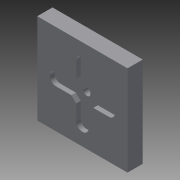
# Autodesk Inventor part: ServoArmTrace
Saved by Autodesk Inventor 2014 (Build 180170000, 170)
## iProperties
Created: 2013-09-20
Part Number: ServoArmTrace
Material: Generic
Document SubType Name: Modeling
Designer: Medrimonia
Density: 1 g/cm^3
Appearance: Default
Author: Medrimonia
Autodesk Inventor part; units mm, degrees
ref_plane "YZ Plane" through (0, 0, 0) normal (1, 0, 0) x (0, 1, 0)
ref_plane "XZ Plane" through (0, 0, 0) normal (0, 1, 0) x (-1, 0, 0)
ref_plane "XY Plane" through (0, 0, 0) normal (0, 0, 1) x (1, 0, 0)
sketch "Sketch1" plane through (0, 0, 0) normal (0, 1, 0) x (-1, 0, 0)
  line L0 (-18.95, -18.95) -> (18.95, -18.95)
  line L1 (18.95, -18.95) -> (18.95, 18.95)
  line L2 (18.95, 18.95) -> (-18.95, 18.95)
  line L3 (-18.95, 18.95) -> (-18.95, -18.95)
  line L4 (-18.95, -18.95) -> (18.95, 18.95) construction
  line L5 (18.95, -18.95) -> (-18.95, 18.95) construction
  line L6 (-2.45, -13.45) -> (2.45, -13.45) construction
  line L7 (2.45, -13.45) -> (2.45, 13.45) construction
  line L8 (2.45, 13.45) -> (-2.45, 13.45) construction
  line L9 (-2.45, 13.45) -> (-2.45, -13.45) construction
  line L10 (-2.45, -13.45) -> (2.45, 13.45) construction
  line L11 (2.45, -13.45) -> (-2.45, 13.45) construction
  line L12 (-13.45, -2.45) -> (13.45, -2.45) construction
  line L13 (13.45, -2.45) -> (13.45, 2.45) construction
  line L14 (13.45, 2.45) -> (-13.45, 2.45) construction
  line L15 (-13.45, 2.45) -> (-13.45, -2.45) construction
  line L16 (-13.45, -2.45) -> (13.45, 2.45) construction
  line L17 (13.45, -2.45) -> (-13.45, 2.45) construction
  line L18 (-13.6, -2.6) -> (13.6, -2.6)
  line L19 (13.6, -2.6) -> (13.6, 2.6)
  line L20 (13.6, 2.6) -> (-13.6, 2.6)
  line L21 (-13.6, 2.6) -> (-13.6, -2.6)
  line L22 (-13.6, -2.6) -> (13.6, 2.6) construction
  line L23 (13.6, -2.6) -> (-13.6, 2.6) construction
  line L24 (-2.6, -13.6) -> (2.6, -13.6)
  line L25 (2.6, -13.6) -> (2.6, 13.6)
  line L26 (2.6, 13.6) -> (-2.6, 13.6)
  line L27 (-2.6, 13.6) -> (-2.6, -13.6)
  line L28 (-2.6, -13.6) -> (2.6, 13.6) construction
  line L29 (2.6, -13.6) -> (-2.6, 13.6) construction
  point P0 (0, 0)
  point P1 (0, 0)
  dimension "d0" = 37.9
  dimension "d1" = 4.9
  dimension "d2" = 11
  dimension "d3" = 0.15
  dimension "d4" = 0.15
  constraints: 60 end point, 12 midpoint, 10 parallel, 10 perpendicular, 5 horizontal
  measures "d0" distance of L1.end L2.end
  measures "d1" distance of L14.end L12.start
  measures "d2" distance between parallel lines of L13 L7
  measures "d3" distance between parallel lines of L25 L7
  measures "d4" distance between parallel lines of L26 L8
extrude "Extrusion1" add sketch "Sketch1" along normal blind 1.9
sketch "Sketch2" plane through (0, 1.9, 0) normal (0, 1, 0) x (1, 0, 0)
  line L0 (18.95, 18.95) -> (-18.95, 18.95) projected
  line L1 (-18.95, 18.95) -> (-18.95, -18.95) projected
  line L2 (-18.95, -18.95) -> (18.95, -18.95) projected
  line L3 (18.95, -18.95) -> (18.95, 18.95) projected
  circle A0 centre (0, 0) radius 1.5
  dimension "d7" = 3
  constraints: 1 centre point, 1 coincident
  measures "d7" diameter of A0
extrude "Extrusion2" add sketch "Sketch2" along normal blind 2
sketch "Sketch3" plane through (0, 3.9, 0) normal (0, 1, 0) x (1, 0, 0)
  circle A0 centre (0, 0) radius 1.5 projected
  line L0 (18.95, 18.95) -> (-18.95, 18.95) projected
  line L1 (-18.95, 18.95) -> (-18.95, -18.95) projected
  line L2 (-18.95, -18.95) -> (18.95, -18.95) projected
  line L3 (18.95, -18.95) -> (18.95, 18.95) projected
  circle A1 centre (0, 0) radius 2.75
  dimension "d10" = 5.5
  constraints: 1 centre point, 1 coincident
  measures "d10" diameter of A1
extrude "Extrusion3" add sketch "Sketch3" along normal blind 2.5 contours L3 L2 L1 L0
chamfer "Chamfer1" distance 2 angle 45 1 edges at (-2.6, 0.95, -2.6)
fillet "Fillet1" radius 2.45 1 edges at (-13.6, 0.95, -2.6)
fillet "Fillet2" radius 2.45 1 edges at (-2.6, 0.95, -13.6)
chamfer "Chamfer2" distance 2 angle 45 1 edges at (2.6, 0.95, -2.6)
chamfer "Chamfer3" distance 2 angle 45 1 edges at (2.6, 0.95, 2.6)
fillet "Fillet3" radius 2.45 1 edges at (13.6, 0.95, -2.6)
fillet "Fillet4" radius 2.45 1 edges at (2.6, 0.95, -13.6)
fillet "Fillet5" radius 2.45 1 edges at (13.6, 0.95, 2.6)
fillet "Fillet6" radius 2.45 1 edges at (2.6, 0.95, 13.6)
chamfer "Chamfer4" distance 2 angle 45 1 edges at (-2.6, 0.95, 2.6)
fillet "Fillet7" radius 2.45 2 edges at (-2.6, 0.95, 13.6) (-13.6, 0.95, 2.6)
equation "\"d0\" = 3 * ServoArmLength + ServoArmWidth"
equation "\"d1\" = ServoArmWidth"
equation "\"d2\" = ServoArmLength"
equation "\"d3\" = ServoArmSpacing"
equation "\"d4\" = ServoArmSpacing"
equation "\"d5\" = ServoArmThickness"
equation "\"d7\" = ServoArmHoleRequired"
equation "\"d8\" = MinimalThickness"
equation "\"d10\" = ServoArmHeadScrewTrace"
equation "\"d11\" = ServoArmHeadScrewThickness"
equation "\"d13\" = ServoArmInternFillet"
equation "\"d16\" = ServoArmExternFillet"
equation "\"d17\" = ServoArmExternFillet"
equation "\"d18\" = ServoArmInternFillet"
equation "\"d21\" = ServoArmInternFillet"
equation "\"d24\" = ServoArmExternFillet"
equation "\"d25\" = ServoArmExternFillet"
equation "\"d26\" = ServoArmExternFillet"
equation "\"d27\" = ServoArmExternFillet"
equation "\"d28\" = ServoArmInternFillet"
equation "\"d31\" = ServoArmExternFillet"
equation "\"ServoArmLength\" = 11"
equation "\"ServoArmWidth\" = 4.9"
equation "\"ServoArmSpacing\" = 0.15"
equation "\"ServoArmThickness\" = 1.9"
equation "\"ServoArmHoleRequired\" = 3"
equation "\"MinimalThickness\" = 2"
equation "\"ServoArmHeadScrewTrace\" = 5.5"
equation "\"ServoArmHeadScrewThickness\" = 2.5"
equation "\"ServoArmInternFillet\" = 2"
equation "\"ServoArmExternFillet\" = 2.45"
body "Solid1"
